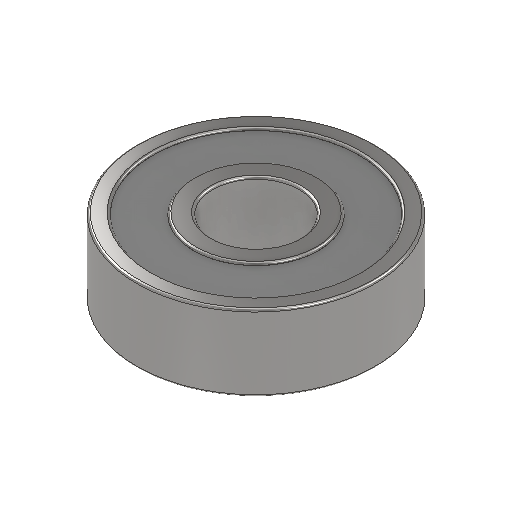
# Autodesk Inventor part: 6082rsBearing
Saved by Autodesk Inventor 2025 (Build 290162000, 162)
## iProperties
Created: 2024-06-25
Part Number: 6082rsBearing
Material: Stainless Steel
Document SubType Name: Modeling
Designer: derm
Density: 8 g/cm^3
Appearance: Semi-Polished
Author: derm
Autodesk Inventor part; units mm, degrees
ref_plane "YZ Plane" through (0, 0, 0) normal (1, 0, 0) x (0, 1, 0)
ref_plane "XZ Plane" through (0, 0, 0) normal (0, 1, 0) x (-1, 0, 0)
sketch "Sketch1" plane through (0, 0, 0) normal (0, 1, 0) x (-1, 0, 0)
  circle A0 centre (0, 0) radius 4
  circle A1 centre (0, 0) radius 11
  dimension "d0" = 22
  dimension "d1" = 8
  constraints: 2 centre point, 2 coincident
  measures "d0" diameter of A1
  measures "d1" diameter of A0
extrude "Extrusion1" add sketch "Sketch1" along normal blind 7
sketch "Sketch2" plane through (0, 7, 0) normal (0, 1, 0) x (1, 0, 0)
  circle A0 centre (0, 0) radius 11 projected
  circle A1 centre (0, 0) radius 4 projected
  circle A2 centre (0, 0) radius 5.75
  circle A3 centre (0, 0) radius 9.5
  dimension "d4" = 19
  dimension "d5" = 11.5
  constraints: 2 centre point, 2 coincident
  measures "d4" diameter of A3
  measures "d5" diameter of A2
extrude "Extrusion2" cut sketch "Sketch2" against normal blind 0.21 contours A3
fillet "Fillet1" radius 0.2 4 edges at (-5.75, 7, 0) (4, 7, 0) (-9.5, 7, 0) (11, 7, 0)
ref_plane "Work Plane1" through (0, 3.5, 0) normal (0, 1, 0) x (1, 0, 0)
mirror "Mirror2" about plane through (0, 3.5, 0) normal (0, 1, 0) of "Extrusion2"
fillet "Fillet2" radius 0.2 4 edges at (-9.5, 0, 0) (11, 0, 0) (-5.75, 0, 0) (4, 0, 0)
body "Solid1"
